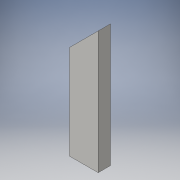
# Autodesk Inventor part: Front Face Bottom Right Support for Slats
Saved by Autodesk Inventor 2016 (Build 200138000, 138)
## iProperties
Created: 2015-07-06
Part Number: Front Face Bottom Right Support for Slats
Material: Generic
Document SubType Name: Modeling
Designer: steele
Density: 1 g/cm^3
Appearance: Default
Author: steele
Autodesk Inventor part; units mm, degrees
ref_plane "YZ Plane" through (0, 0, 0) normal (1, 0, 0) x (0, 1, 0)
ref_plane "XZ Plane" through (0, 0, 0) normal (0, 1, 0) x (-1, 0, 0)
ref_plane "XY Plane" through (0, 0, 0) normal (0, 0, 1) x (1, 0, 0)
sketch "Sketch1" plane through (0, 0, 0) normal (0, 0, 1) x (1, 0, 0)
  line L0 (-48.4973, -207.8455) -> (40.4027, -207.8455)
  line L1 (40.4027, -207.8455) -> (40.4027, 173.1545)
  line L2 (-48.4973, 84.2545) -> (-48.4973, -207.8455)
  line L3 (-48.4973, -207.8455) -> (40.4027, 173.1545) construction
  line L4 (40.4027, -207.8455) -> (18.4243, -94.7809) construction
  line L5 (40.4027, 173.1545) -> (-48.4973, 84.2545)
  line L6 (40.4027, 173.1545) -> (166.1263, 173.1545) construction
  point P0 (0, 0)
  dimension "d1" = 88.9
  dimension "d2" = 381
  dimension "d5" = 45
  constraints: 14 end point, 2 horizontal, 2 point on line, 1 equal length, 1 parallel, 1 perpendicular
  measures "d1" distance of L0.start L0.end
  measures "d2" distance of L0.end L1.end
  measures "d5" angle of L1 L5
extrude "Extrusion1" add sketch "Sketch1" along normal mid plane 38.1
body "Solid1"
